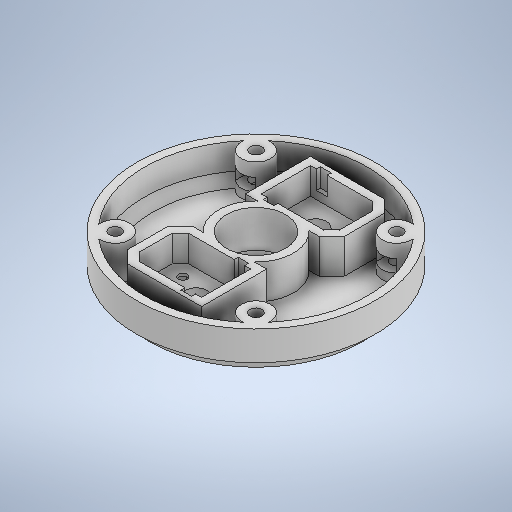
# Autodesk Inventor part: SCARA swivel base - top
Saved by Autodesk Inventor 2025.2 (Build 292293000, 293)
## iProperties
Created: 2025-01-25
Part Number: SCARA swivel base - top
Material: Generic
Document SubType Name: Modeling
Designer: caomi
Density: 1 g/cm^3
Appearance: Default
Author: caomi
Autodesk Inventor part; units mm, degrees
ref_plane "YZ Plane" through (0, 0, 0) normal (1, 0, 0) x (0, 1, 0)
ref_plane "XZ Plane" through (0, 0, 0) normal (0, 1, 0) x (-1, 0, 0)
ref_plane "XY Plane" through (0, 0, 0) normal (0, 0, 1) x (1, 0, 0)
sketch "Sketch1" plane through (0, 0, 0) normal (0, 1, 0) x (-1, 0, 0)
  circle A0 centre (0, 0) radius 45
  line L0 (15.25, 13.25) -> (-11.25, 13.25)
  line L1 (-11.25, 13.25) -> (-11.25, 31.75)
  line L2 (-11.25, 31.75) -> (15.25, 31.75)
  line L3 (42.4598, 22.5) -> (-15.5039, 22.5) construction
  line L4 (0, -63) -> (0, 63) projected
  line L5 (-15.25, -31.75) -> (11.25, -31.75)
  line L6 (11.25, -31.75) -> (11.25, -13.25)
  line L7 (11.25, -13.25) -> (-15.25, -13.25)
  line L8 (19.1191, -22.5) -> (-71.9329, -22.5) construction
  line L9 (68.3866, 0) -> (-95.3195, 0) projected
  circle A1 centre (0, 0) radius 11.1
  circle A2 centre (0, 0) radius 4.5
  line L10 (15.25, 13.25) -> (15.25, 31.75)
  line L11 (-15.25, -13.25) -> (-15.25, -31.75)
  circle A3 centre (9, 26.5) radius 1.65
  circle A4 centre (-9, -26.5) radius 1.65
  line L12 (10.6743, 23.6) -> (7.3257, 23.6)
  line L13 (7.3257, 23.6) -> (5.6514, 26.5)
  line L14 (5.6514, 26.5) -> (7.3257, 29.4)
  line L15 (7.3257, 29.4) -> (10.6743, 29.4)
  line L16 (10.6743, 29.4) -> (12.3486, 26.5)
  line L17 (12.3486, 26.5) -> (10.6743, 23.6)
  line L18 (-5.6514, -26.5) -> (-7.3257, -29.4)
  line L19 (-7.3257, -29.4) -> (-10.6743, -29.4)
  line L20 (-10.6743, -29.4) -> (-12.3486, -26.5)
  line L21 (-12.3486, -26.5) -> (-10.6743, -23.6)
  line L22 (-10.6743, -23.6) -> (-7.3257, -23.6)
  line L23 (-7.3257, -23.6) -> (-5.6514, -26.5)
  circle A5 centre (9, 18.5) radius 1.65
  line L24 (10.6743, 15.6) -> (7.3257, 15.6)
  line L25 (7.3257, 15.6) -> (5.6514, 18.5)
  line L26 (5.6514, 18.5) -> (7.3257, 21.4)
  line L27 (7.3257, 21.4) -> (10.6743, 21.4)
  line L28 (10.6743, 21.4) -> (12.3486, 18.5)
  line L29 (12.3486, 18.5) -> (10.6743, 15.6)
  circle A6 centre (-9, -18.5) radius 1.65
  line L30 (-5.6514, -18.5) -> (-7.3257, -21.4)
  line L31 (-7.3257, -21.4) -> (-10.6743, -21.4)
  line L32 (-10.6743, -21.4) -> (-12.3486, -18.5)
  line L33 (-12.3486, -18.5) -> (-10.6743, -15.6)
  line L34 (-10.6743, -15.6) -> (-7.3257, -15.6)
  line L35 (-7.3257, -15.6) -> (-5.6514, -18.5)
  circle A7 centre (0, 22.5) radius 4.1
  circle A8 centre (0, -22.5) radius 4.1
  point P0 (0, -4.3524)
  dimension "d1" = 18.5
  dimension "d2" = 90
  dimension "d12" = 22.2
  dimension "d26" = 45
  dimension "d50" = 9
  dimension "d53" = 26.5
  dimension "d54" = 15.25
  dimension "d55" = 15.25
  dimension "d56" = 3.3
  dimension "d60" = 5.8
  dimension "d61" = 5.8
  dimension "d70" = 5.8
  dimension "d71" = 8
  dimension "d72" = 5.8
  dimension "d74" = 8
  dimension "d84" = 8.2
  dimension "d89" = 9
  dimension "d90" = 9
  constraints: 68 end point, 9 centre point, 7 horizontal, 7 point on line, 7 vertical alignment, 6 coincident, 4 equal radius, 3 perpendicular, 2 parallel, 2 symmetric about line, 2 vertical, 1 midpoint, 56 other
  measures "d1" distance of L0.end L1.end
  measures "d2" diameter of A0
  measures "d12" diameter of A1
  measures "d26" distance of point (0, 22.5) point (0, -22.5)
  measures "d50" diameter of A2
  measures "d53" distance of L1.end L2.end
  measures "d54" distance from line of L10 point (0, 22.5)
  measures "d55" distance from line of L11 point (0, -22.5)
  measures "d56" diameter of A3
  measures "d60" distance between parallel lines of L12 L15
  measures "d61" distance between parallel lines of L22 L19
  measures "d70" distance between parallel lines of L24 L27
  measures "d71" distance of A5.centre A3.centre
  measures "d72" distance between parallel lines of L34 L31
  measures "d74" distance of A4.centre A6.centre
  measures "d84" diameter of A7
  measures "d89" horizontal distance of A7.centre A3.centre
  measures "d90" horizontal distance of A8.centre A4.centre
extrude "General Shape" add sketch "Sketch1" along normal blind 16 contours L9 A1 L4 L0 L10 L2 A0 | A0 L4 L5 L6 L7 A1 L9 | L4 L2 L1 L0 A1 L9 A0 | A0 L9 A1 L4 L7 L11 L5 | L4 A7 L0 L1 L2 | L2 L10 L0 L4 A7 | L5 L11 L7 L4 A8 | L4 A8 L7 L6 L5 | A7 L4 | L4 A7 | A8 L4 | L4 A8 | A3 | A4 | L12 L13 L14 L15 L16 L17 | L18 L19 L20 L21 L22 L23 | A5 | L24 L25 L26 L27 L28 L29 | A6 | L30 L31 L32 L33 L34 L35
extrude "Shaft support Slot" cut sketch "Sketch1" against normal blind 10 from surface at 16 contours L4 A7 L0 L1 L2 | L2 L10 L0 L4 A7 | L5 L11 L7 L4 A8 | L4 A8 L7 L6 L5 | A7 L4 | L4 A7 | A8 L4 | L4 A8 | A3 | A4 | L12 L13 L14 L15 L16 L17 | L18 L19 L20 L21 L22 L23 | A5 | L24 L25 L26 L27 L28 L29 | A6 | L30 L31 L32 L33 L34 L35
chamfer "Corners of shaft support slots" distance 3 angle 45 4 edges at (-15.25, 11, 31.75) (-15.25, 11, 13.25) (15.25, 11, -13.25) (15.25, 11, -31.75)
extrude "T3 nut slots" cut sketch "Sketch1" along normal blind 5 contours A3 | A4 | L12 L13 L14 L15 L16 L17 | L18 L19 L20 L21 L22 L23 | A5 | L24 L25 L26 L27 L28 L29 | A6 | L30 L31 L32 L33 L34 L35
extrude "Holes for smooth rod & M3 bolt" cut sketch "Sketch1" along normal up to surface (6 mm away) contours A7 L4 | L4 A7 | A8 L4 | L4 A8 | A3 | A4 | A5 | A6
extrude "Base for 608 Bearing" add sketch "Sketch1" along normal blind 2 contours A1 L4 A2 L9 | L9 A2 L4 A1 | L4 A2 L9 A1 | A1 L9 A2 L4
chamfer "Material reduction on the base" distance 5 angle 45 1 edges at (45, 0, 0)
shell "Shell1" thickness 3 removed faces 1 at (23.348, 16, -9.4208)
sketch "Sketch4" plane through (0, 16, 0) normal (0, 1, 0) x (1, 0, 0)
  circle A0 centre (-26.5165, -26.5165) radius 2.25
  line L0 (0, 0) -> (-69.9236, 0) construction
  line L1 (-26.5165, -26.5165) -> (0, 0) construction
  line L2 (-30.2665, -28.6816) -> (-30.2665, -24.3514)
  line L3 (-30.2665, -24.3514) -> (-26.5165, -22.1864)
  line L4 (-26.5165, -22.1864) -> (-22.7665, -24.3514)
  line L5 (-22.7665, -24.3514) -> (-22.7665, -28.6816)
  line L6 (-22.7665, -28.6816) -> (-26.5165, -30.8466)
  line L7 (-26.5165, -30.8466) -> (-30.2665, -28.6816)
  circle A1 centre (-26.5165, -26.5165) radius 5.5
  line L8 (-30.2665, -24.3514) -> (-30.2665, -22.4931)
  line L9 (-22.7665, -24.3514) -> (-22.7665, -22.4931)
  circle A2 centre (-26.5165, 26.5165) radius 2.25
  line L10 (-30.2665, 28.6816) -> (-30.2665, 24.3514)
  line L11 (-30.2665, 24.3514) -> (-26.5165, 22.1864)
  line L12 (-26.5165, 22.1864) -> (-22.7665, 24.3514)
  line L13 (-22.7665, 24.3514) -> (-22.7665, 28.6816)
  line L14 (-22.7665, 28.6816) -> (-26.5165, 30.8466)
  line L15 (-26.5165, 30.8466) -> (-30.2665, 28.6816)
  circle A3 centre (-26.5165, 26.5165) radius 5.5
  line L16 (-30.2665, 24.3514) -> (-30.2665, 22.4931)
  line L17 (-22.7665, 24.3514) -> (-22.7665, 22.4931)
  line L18 (0, -9.8059) -> (0, 7.3238) construction
  circle A4 centre (26.5165, -26.5165) radius 2.25
  line L19 (30.2665, -28.6816) -> (30.2665, -24.3514)
  line L20 (30.2665, -24.3514) -> (26.5165, -22.1864)
  line L21 (26.5165, -22.1864) -> (22.7665, -24.3514)
  line L22 (22.7665, -24.3514) -> (22.7665, -28.6816)
  line L23 (22.7665, -28.6816) -> (26.5165, -30.8466)
  line L24 (26.5165, -30.8466) -> (30.2665, -28.6816)
  circle A5 centre (26.5165, -26.5165) radius 5.5
  line L25 (30.2665, -24.3514) -> (30.2665, -22.4931)
  line L26 (22.7665, -24.3514) -> (22.7665, -22.4931)
  circle A6 centre (26.5165, 26.5165) radius 2.25
  line L27 (30.2665, 24.3514) -> (26.5165, 22.1864)
  line L28 (26.5165, 22.1864) -> (22.7665, 24.3514)
  line L29 (22.7665, 24.3514) -> (22.7665, 28.6816)
  line L30 (22.7665, 28.6816) -> (26.5165, 30.8466)
  circle A7 centre (26.5165, 26.5165) radius 5.5
  line L31 (30.2665, 24.3514) -> (30.2665, 22.4931)
  line L32 (22.7665, 24.3514) -> (22.7665, 22.4931)
  line L33 (26.5165, 30.8466) -> (30.2665, 28.6816)
  line L34 (30.2665, 28.6816) -> (30.2665, 24.3514)
  dimension "d32" = 4.5
  dimension "d44" = 37.5
  dimension "d76" = 45
  dimension "d77" = 7.5
  dimension "d78" = 11
  constraints: 70 end point, 33 symmetric about line, 9 coincident, 8 centre point, 8 point on circle, 2 collinear, 2 vertical, 1 horizontal, 1 point on line, 19 other
  measures "d32" diameter of A0
  measures "d44" distance of L1.start point (0, 0)
  measures "d76" angle of L1 L0
  measures "d77" distance between parallel lines of L5 L2
  measures "d78" diameter of A1
extrude "Slot for M4 fasteners" add sketch "Sketch4" against normal up to surface (13 mm away)
ref_plane "Work Plane4" through (0, 11, 0) normal (0, 1, 0) x (1, 0, 0)
extrude "Slot for M4 nuts to fasen to the swivel base" cut sketch "Sketch4" against normal blind 4.7 from surface at -5 contours L2 L3 L4 L5 L6 L7 | L8 A1 L9 L4 L3 | L15 L14 L13 L12 L11 L10 | L11 L12 L17 A3 L16 | L24 L23 L22 L21 L20 L19 | L20 L21 L26 A5 L25 | L31 A7 L32 L28 L27 | L27 L28 L29 L30 L33 L34
sketch "Sketch6" plane through (0, 16, 0) normal (0, 1, 0) x (1, 0, 0)
  line L0 (9, -11.75) -> (5, -11.75)
  line L1 (5, -11.75) -> (5, -33.25)
  line L2 (5, -33.25) -> (9, -33.25)
  line L3 (9, -33.25) -> (9, -11.75)
  line L4 (9, -11.75) -> (5, -33.25) construction
  line L5 (5, -11.75) -> (9, -33.25) construction
  circle A0 centre (0, -22.5) radius 4.1 projected
  point P0 (0, 0)
  point P1 (7, -22.5)
  dimension "d94" = 4
  dimension "d95" = 7
  dimension "d96" = 21.5
  constraints: 12 end point, 2 midpoint, 2 parallel, 1 horizontal, 1 horizontal alignment, 1 perpendicular
  measures "d94" distance between parallel lines of L3 L1
  measures "d95" distance of A0.centre point (7, -22.5)
  measures "d96" distance of L2.end L0.start
extrude "Extrusion13" cut sketch "Sketch6" against normal blind 7 contours L3 L2 L1 L0
pattern_circular "Circular Pattern2" count 2 over 360 about axis through (0, 0, 0) along (0, 1, 0) of "Extrusion13"
body "Solid1"
